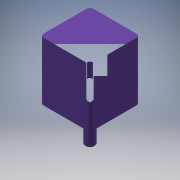
# Autodesk Inventor part: Nema 11
Saved by Autodesk Inventor 2016 (Build 200138000, 138)
## iProperties
Created: 2015-07-20
Part Number: Nema 11
Material: Generic
Document SubType Name: Modeling
Designer: bastli
Density: 1 g/cm^3
Appearance: Violet
Author: bastli
Autodesk Inventor part; units mm, degrees
ref_plane "YZ Plane" through (0, 0, 0) normal (1, 0, 0) x (0, 1, 0)
ref_plane "XZ Plane" through (0, 0, 0) normal (0, 1, 0) x (-1, 0, 0)
ref_plane "XY Plane" through (0, 0, 0) normal (0, 0, 1) x (1, 0, 0)
derived "Fixture.ipt"
sketch "Sketch1" plane through (0, 0, 0) normal (0, 0, 1) x (1, 0, 0)
  line L0 (-14.15, 14.15) -> (14.15, 14.15)
  line L1 (14.15, 14.15) -> (14.15, -14.15)
  line L2 (14.15, -14.15) -> (-14.15, -14.15)
  line L3 (-14.15, -14.15) -> (-14.15, 14.15)
  line L4 (-14.15, 14.15) -> (14.15, -14.15) construction
  line L5 (14.15, 14.15) -> (-14.15, -14.15) construction
  circle A0 centre (0, 0) radius 11
  line L6 (-11.5, -11.5) -> (11.5, -11.5)
  line L7 (11.5, -11.5) -> (11.5, 11.5)
  line L8 (11.5, 11.5) -> (-11.5, 11.5)
  line L9 (-11.5, 11.5) -> (-11.5, -11.5)
  line L10 (-11.5, -11.5) -> (11.5, 11.5) construction
  line L11 (11.5, -11.5) -> (-11.5, 11.5) construction
  point P0 (0, 0)
  dimension "d0" = 28.3
  dimension "d2" = 22
  dimension "d22" = 23
  constraints: 24 end point, 5 coincident, 4 midpoint, 4 parallel, 3 perpendicular, 2 horizontal, 1 centre point, 1 point on line
  measures "d0" distance of L0.start L0.end
  measures "d2" diameter of A0
  measures "d22" distance of L7.end L8.end
extrude "Extrusion1" add sketch "Sketch1" along normal blind 51 contours L0 L1 L2 L3 | A0 | L9 L8 L7 L6
sketch "Sketch4" plane through (0, 0, 0) normal (0, 0, -1) x (-1, 0, 0)
  point P0 (0, 0)
  point P1 (11.5, -11.5)
  point P2 (-11.5, -11.5)
  point P3 (-11.5, 11.5)
  point P4 (11.5, 11.5)
hole "Hole2" at (11.5, -11.5, 0) at (-11.5, -11.5, 0) at (-11.5, 11.5, 0) at (11.5, 11.5, 0) direction (0, 0, 1) diameter 2.5 depth 8 tip angle 118
sketch "Sketch3" plane through (0, 0, 0) normal (0, 0, -1) x (-1, 0, 0)
  circle A0 centre (0, 0) radius 2.65
  circle A1 centre (0, 0) radius 11
  dimension "d30" = 22
  dimension "d31" = 5.3
  constraints: 2 centre point, 2 coincident
  measures "d30" diameter of A1
  measures "d31" diameter of A0
extrude "Extrusion2" add sketch "Sketch3" along normal blind 2 contours A0 | A1
extrude "Extrusion3" add sketch "Sketch3" along normal blind 20 contours A0
chamfer "Chamfer1" distance 0.6 angle 45 1 edges at (2.65, 0, -20)
fillet "Fillet1" radius 2.16 4 edges at (-14.15, -14.15, 25.5) (-14.15, 14.15, 25.5) (14.15, -14.15, 25.5) (14.15, 14.15, 25.5)
equation "\"d0\" = nema_11_width"
equation "\"d2\" = nema_11_foot_diameter"
equation "\"d22\" = nema_11_hole_distance"
equation "\"d3\" = nema_11_length"
equation "\"d30\" = nema_11_foot_diameter"
equation "\"d31\" = nema_11_transmission_radius"
equation "\"d12\" = nema_11_transmission_foot"
equation "\"d15\" = nema_11_transmission_length"
equation "\"nema_11_width\" = 28.3"
equation "\"nema_11_foot_diameter\" = 22"
equation "\"nema_11_hole_distance\" = 23"
equation "\"nema_11_length\" = 51"
equation "\"nema_11_transmission_radius\" = 5.3"
equation "\"nema_11_transmission_foot\" = 2"
equation "\"nema_11_transmission_length\" = 20"
body "Solid1"
